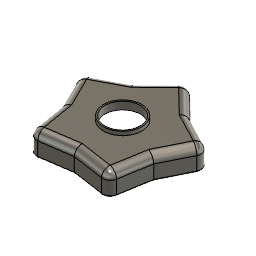
Star Lid (Autodesk Fusion 360 archive; units mm, degrees)
design "Star"
part number: 2026-06-13-20-13-12-227
Autodesk Fusion 360 part; units mm, degrees
note: some values were not read from the file. Set by a fixed rule: which face or edge a step refers to.
sketch "Sketch1" plane through (0, 0, 0) normal (0, 1, 0) x (1, 0, 0)
  line L0 (0, 80) -> (-33.9737, 46.7608)
  line L1 (0, 80) -> (33.9737, 46.7608)
  line L2 (-76.0845, 24.7214) -> (-33.9737, 46.7608)
  line L3 (-76.0845, 24.7214) -> (-54.9706, -17.861)
  line L4 (-47.0228, -64.7214) -> (-54.9706, -17.861)
  line L5 (-47.0228, -64.7214) -> (0, -57.7996)
  line L6 (47.0228, -64.7214) -> (0, -57.7996)
  line L7 (47.0228, -64.7214) -> (54.9706, -17.861)
  line L8 (76.0845, 24.7214) -> (54.9706, -17.861)
  line L9 (76.0845, 24.7214) -> (33.9737, 46.7608)
  circle A0 centre (0, 0) radius 25
  dimension "d35" = 50
  constraint coincident A0.centre origin
  measures "d35" diameter of A0
extrude "Extrude1" add sketch "Sketch1" along normal blind 25 contours L0 L1 L2 L3 L4 L5 L6 L7 L8 L9 | A0 makes body 1
shell "Shell1" thickness 5 outward yes removed faces 1 at (11.3246, 25, -3.6796) on bodies 1
extrude "Extrude2" add 1 faces at (-65.2553, 25, -34.1513) along direction (0, 1, 0) blind 5 separate body on bodies 1 makes body 2
extrude "Extrude3" add sketch "Sketch1" along normal blind 30 separate body contours L0 L1 L2 L3 L4 L5 L6 L7 L8 L9 | A0 makes body 3
extrude "Extrude4" cut 1 faces at (11.3246, 0, -3.6796) along direction (0, 1, 0) blind 25 on bodies 3 bodies 3
sketch "Sketch2" plane through (0, 30, 0) normal (0, 1, 0) x (-1, 0, 0)
  line L0 (-47.0228, 64.7214) -> (-54.9706, 17.861)
  line L1 (-54.9706, 17.861) -> (-76.0845, -24.7214)
  line L2 (-76.0845, -24.7214) -> (-33.9737, -46.7608)
  line L3 (-33.9737, -46.7608) -> (0, -80)
  line L4 (0, -80) -> (33.9737, -46.7608)
  line L5 (33.9737, -46.7608) -> (76.0845, -24.7214)
  line L6 (76.0845, -24.7214) -> (54.9706, 17.861)
  line L7 (54.9706, 17.861) -> (47.0228, 64.7214)
  line L8 (47.0228, 64.7214) -> (0, 57.7996)
  line L9 (0, 57.7996) -> (-47.0228, 64.7214)
  circle A0 centre (0, 0) radius 25
  dimension "d65" = 50
  constraint coincident A0.centre origin
  measures "d65" diameter of A0
extrude "Extrude9" cut sketch "Sketch1" against normal blind 10 bodies 1 makes body 4 at (-6.7759, 0, 1.242)
extrude "Extrude10" cut 1 faces at (-6.7759, -5, 1.242) along direction (0, 1, 0) blind 10 on bodies 4 bodies 4
delete_body "RemoveBody1" bodies 4
extrude "Extrude14" cut sketch "Sketch2" against normal blind 5 contours A0 bodies 3
extrude "Extrude15" add sketch "Sketch2" along normal blind 5 separate body contours A0 makes body 5
shell "Shell5" thickness 2 removed faces 1 at (6.7759, 35, -1.242) on bodies 5
extrude "Extrude16" cut 1 faces at (-4.7801, 32, 5.994) along direction (0, -1, 0) blind 10 on bodies 5 bodies 5
extrude "Extrude17" add 1 faces at (-24.1546, 30, -2.3847) along direction (0, -1, 0) blind 5 on bodies 5 bodies 3 5
combine "Combine1" operation add target body 2 tool bodies 1 3
fillet "Fillet1" radius 10 5 edges at (-51.1344, 12.5, 70.3805) (-82.7372, 12.5, -26.8829) (0, 12.5, -86.995) (82.7372, 12.5, -26.8829) (51.1344, 12.5, 70.3805) on bodies 2
extrude "Extrude18" cut 1 faces at (29.4926, -5, 63.8255) along direction (0, 1, 0) blind 5 on bodies 2 bodies 2
fillet "Fillet2" radius 10 15 edges at (56.2738, 30, 40.0786) (48.7891, 30, 67.1524) (20.7275, 30, 65.9045) (55.5066, 30, -41.1346) (78.9424, 30, -25.6499) (69.0841, 30, 0.6526) (-21.9688, 30, -65.5012) (0, 30, -83.005) (21.9688, 30, -65.5012) (-69.0841, 30, 0.6526) (-78.9424, 30, -25.6499) (-55.5066, 30, -41.1346) (-20.7275, 30, 65.9045) (-48.7891, 30, 67.1524) (-56.2738, 30, 40.0786) on bodies 2
fillet "Fillet3" radius 2.5 15 edges at (69.0841, 0, 0.6526) (78.9424, 0, -25.6499) (55.5066, 0, -41.1346) (21.9688, 0, -65.5012) (0, 0, -83.005) (-21.9688, 0, -65.5012) (-55.5066, 0, -41.1346) (-78.9424, 0, -25.6499) (-69.0841, 0, 0.6526) (-56.2738, 0, 40.0786) (-48.7891, 0, 67.1524) (-20.7275, 0, 65.9045) (20.7275, 0, 65.9045) (48.7891, 0, 67.1524) (56.2738, 0, 40.0786) on bodies 2
extrude "Extrude19" add sketch "Sketch1" along normal blind 5 separate body makes body 6
extrude "Extrude20" add sketch "Sketch1" along normal blind 5 contours A0 bodies 6
shell "Shell6" thickness 2 removed faces 1 at (11.3246, 5, -3.6796) on bodies 6
hidden bodies 6
